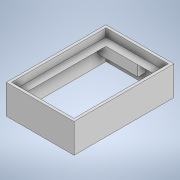
# Autodesk Inventor part: sensorCover
Saved by Autodesk Inventor 2022 (Build 260153000, 153)
## iProperties
Created: 2023-11-20
Part Number: sensorCover
Material: Generic
Document SubType Name: Modeling
Designer: Timber
Density: 1 g/cm^3
Appearance: Default
Author: Timber
Autodesk Inventor part; units mm, degrees
ref_plane "YZ Plane" through (0, 0, 0) normal (1, 0, 0) x (0, 1, 0)
ref_plane "XZ Plane" through (0, 0, 0) normal (0, 1, 0) x (-1, 0, 0)
ref_plane "XY Plane" through (0, 0, 0) normal (0, 0, 1) x (1, 0, 0)
sketch "Sketch1" plane through (0, 0, 0) normal (0, 1, 0) x (-1, 0, 0)
  line L0 (0, 0) -> (23, 0) construction
  line L1 (23, 0) -> (23, -35) construction
  line L2 (23, -35) -> (0, -35) construction
  line L3 (0, -35) -> (0, 0) construction
  line L4 (23.25, -35.25) -> (23.25, 0.25)
  line L5 (23.25, 0.25) -> (-0.25, 0.25)
  line L6 (-0.25, 0.25) -> (-0.25, -35.25)
  line L7 (-0.25, -35.25) -> (23.25, -35.25)
  line L8 (24.25, 1.25) -> (24.25, -36.25)
  line L9 (24.25, -36.25) -> (-1.25, -36.25)
  line L10 (-1.25, -36.25) -> (-1.25, 1.25)
  line L11 (-1.25, 1.25) -> (24.25, 1.25)
  dimension "d0" = 35
  dimension "d1" = 23
  dimension "d2" = 0.25
  dimension "d3" = 1
  constraints: 24 end point, 6 parallel, 3 perpendicular, 1 horizontal, 6 other
  measures "d0" distance of L0.end L1.end
  measures "d1" distance of L1.end L2.end
  measures "d2" distance between parallel lines of L1 L4
  measures "d3" distance between parallel lines of L4 L8
extrude "Extrusion1" add sketch "Sketch1" along normal blind 8
sketch "Sketch9" plane through (0.25, 0, 0.25) normal (0, 0, -1) x (-1, 0, 0)
  line L0 (-1, 0) -> (24.5, 0) projected
  line L1 (24.5, 0) -> (24.5, 8) projected
  line L2 (-1, 8) -> (24.5, 8) projected
  line L3 (-1, 0) -> (-1, 8) projected
  line L4 (0, 0) -> (23.5, 0) projected
  line L5 (23.5, 0) -> (23.5, 8) projected
  line L6 (0, 8) -> (23.5, 8) projected
  line L7 (0, 0) -> (0, 8) projected
  line L8 (0, 8) -> (3, 8)
  line L9 (24.5, 8) -> (-1, 8) projected
  line L10 (3, 8) -> (0, 5.5)
  line L11 (0, 0) -> (0, 8) projected
  line L12 (0, 8) -> (0, 5.5)
  point P0 (0.25, 0)
  point P1 (0, 8)
  dimension "d25" = 3
  dimension "d26" = 2.5
  constraints: 6 end point, 2 point on line, 1 collinear
  measures "d25" distance of L6.start L8.end
  measures "d26" distance of L6.start L10.end
extrude "Extrusion7" add sketch "Sketch9" along normal up to surface (35.5 mm away) contours L7 L2 L10
ref_plane "Work Plane5" through (-11.5, 0, 1.25) normal (1, 0, 0) x (0, 0, -1)
mirror "Mirror4" about plane through (-11.5, 0, 1.25) normal (1, 0, 0) of "Extrusion7"
sketch "Sketch10" plane through (0.25, 0, -35.25) normal (-1, 0, 0) x (0, 0, 1)
  line L0 (-1, 0) -> (36.5, 0) projected
  line L1 (36.5, 0) -> (36.5, 8) projected
  line L2 (-1, 8) -> (36.5, 8) projected
  line L3 (-1, 0) -> (-1, 8) projected
  line L4 (35.5, 5.5) -> (0, 5.5) projected
  line L5 (0, 0) -> (0, 5.5) projected
  line L6 (0, 0) -> (35.5, 0) projected
  line L7 (35.5, 0) -> (35.5, 5.5) projected
  line L8 (36.5, 8) -> (-1, 8) projected
  line L9 (0, 8) -> (3, 8)
  line L10 (0, 0) -> (0, 5.5) projected
  line L11 (3, 8) -> (0, 5.5)
  line L12 (35.5, 5.5) -> (0, 5.5) projected
  line L13 (0, 8) -> (0, 5.5)
  point P0 (35.25, 0)
  point P1 (3, 8)
  dimension "d29" = 3
  constraints: 6 end point, 2 point on line, 1 vertical
  measures "d29" distance of L9.start L9.end
extrude "Extrusion8" add sketch "Sketch10" along normal up to surface (23.5 mm away) contours L13 L2 L11
ref_plane "Work Plane6" through (-24.25, 0, -17.5) normal (0, 0, 1) x (1, 0, 0)
mirror "Mirror5" about plane through (-24.25, 0, -17.5) normal (0, 0, 1) of "Extrusion8"
sketch "Sketch11" plane through (0, 8, 0) normal (0, 1, 0) x (1, 0, 0)
  line L0 (1.25, -1.25) -> (1.25, 36.25) projected
  line L1 (-24.25, -1.25) -> (1.25, -1.25) projected
  line L2 (-24.25, 36.25) -> (-24.25, -1.25) projected
  line L3 (1.25, 36.25) -> (-24.25, 36.25) projected
  line L4 (-23.25, 35.25) -> (0.25, 35.25) projected
  line L5 (-23.25, -0.25) -> (-23.25, 35.25) projected
  line L6 (0.25, -0.25) -> (-23.25, -0.25) projected
  line L7 (0.25, 35.25) -> (0.25, -0.25) projected
  point P0 (0, 0)
extrude "Extrusion9" add sketch "Sketch11" along normal blind 3
sketch "Sketch12" plane through (-23.25, 0, -35.25) normal (0, 0, 1) x (1, 0, 0)
  line L0 (23.5, 5.5) -> (0, 5.5) projected
  line L1 (0, 0) -> (0, 5.5) projected
  line L2 (0, 0) -> (23.5, 0) projected
  line L3 (23.5, 0) -> (23.5, 5.5) projected
  line L4 (0, 5.5) -> (15, 5.5)
  line L5 (15, 5.5) -> (15, 3.5)
  line L6 (15, 3.5) -> (0, 3.5)
  line L7 (0, 3.5) -> (0, 5.5)
  point P0 (23.25, 0)
  point P1 (0, 5.5)
  point P2 (0, 3.5)
  dimension "d34" = 3.5
  dimension "d35" = 2
  dimension "d36" = 15
  constraints: 8 end point, 2 parallel, 1 collinear, 1 horizontal, 1 perpendicular
  measures "d34" distance between parallel lines of L2 L6
  measures "d35" distance of L4.end L5.end
  measures "d36" distance of L4.start L4.end
extrude "Extrusion10" add sketch "Sketch12" along normal blind 3 contours L5 L6 L1 L0
sketch "Sketch13" plane through (0.25, 0, 0.25) normal (0, 0, -1) x (-1, 0, 0)
  line L0 (23.5, 3.5) -> (23.5, 5.5) projected
  line L1 (8.5, 5.5) -> (23.5, 5.5) projected
  line L2 (8.5, 3.5) -> (23.5, 3.5) projected
  line L3 (23.5, 0) -> (23.5, 3.5) projected
  line L4 (23.5, 0) -> (0, 0) projected
  line L5 (0, 0) -> (0, 5.5) projected
  line L6 (0, 5.5) -> (8.5, 5.5) projected
  line L7 (8.5, 5.5) -> (8.5, 3.5) projected
  line L8 (7.5, 5.5) -> (7.5, 3.5)
  line L9 (7.5, 3.5) -> (3.5, 3.5)
  line L10 (3.5, 3.5) -> (3.5, 5.5)
  line L11 (3.5, 5.5) -> (7.5, 5.5)
  line L12 (21.5, 5.5) -> (23.5, 5.5)
  line L13 (23.5, 5.5) -> (23.5, 3.5)
  line L14 (23.5, 3.5) -> (21.5, 3.5)
  line L15 (21.5, 3.5) -> (21.5, 5.5)
  point P0 (0.25, 0)
  dimension "d40" = 4
  dimension "d41" = 2
  dimension "d42" = 3.5
  dimension "d49" = 2
  constraints: 16 end point, 4 parallel, 3 collinear, 3 perpendicular, 1 horizontal, 1 point on line
  measures "d40" distance of L10.end L8.start
  measures "d41" distance of L8.start L8.end
  measures "d42" distance between parallel lines of L10 L5
  measures "d49" distance between parallel lines of L0 L15
extrude "Extrusion11" add sketch "Sketch13" along normal blind 2 contours L2 L15 L1 L0 | L8 L9 L10 L6
sketch "Sketch18" plane through (-23.25, 5.5, -35.25) normal (0, 1, 0) x (1, 0, 0)
  line L0 (16, -35.5) -> (20, -35.5) projected
  line L1 (20, -35.5) -> (20, -33.5) projected
  line L2 (16, -33.5) -> (20, -33.5) projected
  line L3 (16, -35.5) -> (16, -33.5) projected
  line L4 (0, -35.5) -> (2, -35.5) projected
  line L5 (2, -35.5) -> (2, -33.5) projected
  line L6 (0, -33.5) -> (2, -33.5) projected
  line L7 (0, -33.5) -> (0, -35.5) projected
  line L8 (15, 0) -> (0, 0) projected
  line L9 (0, 0) -> (0, -3) projected
  line L10 (15, -3) -> (0, -3) projected
  line L11 (15, 0) -> (15, -3) projected
  point P0 (23.25, -35.25)
extrude "Extrusion14" add sketch "Sketch18" along normal up to surface (2.5 mm away)
sketch "Sketch20" plane through (-23.25, 3.5, -35.25) normal (0, -1, 0) x (1, 0, 0)
  line L0 (0, 35.5) -> (2, 35.5) projected
  line L1 (0, 33.5) -> (0, 35.5) projected
  line L2 (2, 33.5) -> (0, 33.5) projected
  line L3 (2, 35.5) -> (2, 33.5) projected
  line L4 (16, 35.5) -> (20, 35.5) projected
  line L5 (16, 35.5) -> (16, 33.5) projected
  line L6 (20, 33.5) -> (16, 33.5) projected
  line L7 (20, 35.5) -> (20, 33.5) projected
  line L8 (15, 0) -> (0, 0) projected
  line L9 (15, 0) -> (15, 3) projected
  line L10 (0, 3) -> (15, 3) projected
  line L11 (0, 0) -> (0, 3) projected
  point P0 (23.25, 35.25)
extrude "Extrusion16" cut sketch "Sketch20" against normal blind 0.5
sketch "Sketch22" plane through (-23.25, 0, -35.25) normal (0, 0, 1) x (1, 0, 0)
  point P0 (23.25, 0)
sketch "Sketch23" plane through (-23.25, 0, -35.25) normal (0, 0, 1) x (1, 0, 0)
  point P0 (23.25, 0)
body "Solid1"
